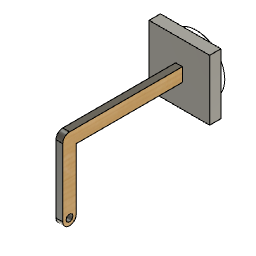
stamp1 v4 (Autodesk Fusion 360 design; units mm, degrees)
Autodesk Fusion 360 part; units mm, degrees
note: some values were not read from the file. Chosen so that the rebuilt part matches the saved one: which bodies a step acts on.
sketch "Sketch1" plane through (0, 0, 0) normal (0, 1, 0) x (1, 0, 0)
  arc A0 (0.3848, -1.12) -> (0.9072, -0.7632) centre (-0.0957, 0.1445) ccw
  arc A1 (3.1397, -0.683) -> (4.2167, 0.662) centre (1.059, 2.0869) ccw
  arc A2 (0.9072, -0.7632) -> (2.7383, -0.9246) centre (1.9676, 0.8001) ccw
  arc A3 (3.0458, -0.7511) -> (3.0474, -0.7499) centre (2.7604, -0.3405) ccw
  arc A4 (-1.811, -5.1195) -> (0.4336, -3.2886) centre (-2.5419, -1.932) ccw
  arc A5 (3.5281, -4.1281) -> (3.0649, -1.2688) centre (0.4022, -3.1674) ccw
  arc A6 (1.1624, -0.2268) -> (1.1146, 0.4041) centre (-0.173, -0.0107) ccw
  arc A7 (1.1146, 0.4041) -> (2.1699, 1.9092) centre (0.2909, 2.1041) ccw
  arc A8 (5.3391, 0.9914) -> (2.6312, 2.0198) centre (2.9441, -1.2354) ccw
  arc A9 (0.7776, 0.8933) -> (0.2074, 1.1673) centre (-0.0773, -0.1552) ccw
  arc A10 (0.2074, 1.1673) -> (-0.5684, 2.8338) centre (-1.6767, 1.304) ccw
  arc A11 (-0.9784, 3.0605) -> (-2.6817, 3.3207) centre (-2.3368, -0.1263) ccw
  arc A12 (1.811, 5.1195) -> (-0.4336, 3.2886) centre (2.5419, 1.932) ccw
  arc A13 (-0.3848, 1.12) -> (-0.9072, 0.7632) centre (0.0957, -0.1445) ccw
  arc A14 (-0.9072, 0.7632) -> (-2.7383, 0.9246) centre (-1.9676, -0.8001) ccw
  arc A15 (-3.1397, 0.683) -> (-4.2167, -0.662) centre (-1.059, -2.0869) ccw
  arc A16 (-3.5281, 4.1281) -> (-3.0649, 1.2688) centre (-0.4022, 3.1674) ccw
  arc A17 (-1.1624, 0.2268) -> (-1.1146, -0.4041) centre (0.173, 0.0107) ccw
  arc A18 (-1.1146, -0.4041) -> (-2.1699, -1.9092) centre (-0.2909, -2.1041) ccw
  arc A19 (-2.1613, -2.3776) -> (-1.535, -3.9828) centre (1.2778, -1.9605) ccw
  arc A20 (-5.3391, -0.9914) -> (-2.6312, -2.0198) centre (-2.9441, 1.2354) ccw
  arc A21 (-0.7776, -0.8933) -> (-0.2074, -1.1673) centre (0.0773, 0.1552) ccw
  arc A22 (-0.2074, -1.1673) -> (0.5684, -2.8338) centre (1.6767, -1.304) ccw
  arc A23 (0.9784, -3.0605) -> (2.6817, -3.3207) centre (2.3368, 0.1263) ccw
  arc A24 (0.5684, -2.8338) -> (0.3848, -1.12) centre (-2.2605, -2.2702) ccw
  arc A25 (-2.1699, -1.9092) -> (-0.7776, -0.8933) centre (-3.0963, 0.8225) ccw
  arc A26 (-2.7383, 0.9246) -> (-1.1624, 0.2268) centre (-0.8358, 3.0927) ccw
  arc A27 (-0.5684, 2.8338) -> (-0.3848, 1.12) centre (2.2605, 2.2702) ccw
  arc A28 (2.1699, 1.9092) -> (0.7776, 0.8933) centre (3.0963, -0.8225) ccw
  arc A29 (2.7383, -0.9246) -> (1.1624, -0.2268) centre (0.8358, -3.0927) ccw
  line L0 (6.7, -6.7) -> (-6.7, -6.7)
  line L1 (-6.7, -6.7) -> (-6.7, 6.7)
  line L2 (-6.7, 6.7) -> (6.7, 6.7)
  line L3 (6.7, 6.7) -> (6.7, -6.7)
  arc A30 (-0.6739, -1.5178) -> (0.4336, -3.2886) centre (1.5858, -1.3364) ccw
  arc A31 (0.818, -3.4693) -> (2.6817, -3.3207) centre (1.5858, -1.3364) ccw
  arc A32 (-1.811, -5.1195) -> (0.818, -3.4693) centre (-1.8093, -2.2029) ccw
  arc A33 (0.9784, -3.0605) -> (0.9775, -1.3425) centre (-1.8093, -2.2029) ccw
  arc A34 (0.9775, -1.3425) -> (3.0649, -1.2688) centre (1.9502, 0.7051) ccw
  arc A35 (3.4135, -1.0262) -> (4.2167, 0.662) centre (1.9502, 0.7051) ccw
  arc A36 (3.1397, -0.683) -> (1.6513, 0.1753) centre (1.0032, -2.6683) ccw
  arc A37 (3.5281, -4.1281) -> (3.4135, -1.0262) centre (1.0032, -2.6683) ccw
  arc A38 (1.6513, 0.1753) -> (2.6312, 2.0198) centre (0.3645, 2.0415) ccw
  arc A39 (2.5955, 2.4431) -> (1.535, 3.9828) centre (0.3645, 2.0415) ccw
  arc A40 (2.1613, 2.3776) -> (0.6739, 1.5178) centre (2.8124, -0.4654) ccw
  arc A41 (5.3391, 0.9914) -> (2.5955, 2.4431) centre (2.8124, -0.4654) ccw
  arc A42 (0.6739, 1.5178) -> (-0.4336, 3.2886) centre (-1.5858, 1.3364) ccw
  arc A43 (-0.818, 3.4693) -> (-2.6817, 3.3207) centre (-1.5858, 1.3364) ccw
  arc A44 (-0.9784, 3.0605) -> (-0.9775, 1.3425) centre (1.8093, 2.2029) ccw
  arc A45 (1.811, 5.1195) -> (-0.818, 3.4693) centre (1.8093, 2.2029) ccw
  arc A46 (-0.9775, 1.3425) -> (-3.0649, 1.2688) centre (-1.9502, -0.7051) ccw
  arc A47 (-3.4135, 1.0262) -> (-4.2167, -0.662) centre (-1.9502, -0.7051) ccw
  arc A48 (-3.1397, 0.683) -> (-1.6513, -0.1753) centre (-1.0032, 2.6683) ccw
  arc A49 (-3.5281, 4.1281) -> (-3.4135, 1.0262) centre (-1.0032, 2.6683) ccw
  arc A50 (-1.6513, -0.1753) -> (-2.6312, -2.0198) centre (-0.3645, -2.0415) ccw
  arc A51 (-2.5955, -2.4431) -> (-1.535, -3.9828) centre (-0.3645, -2.0415) ccw
  arc A52 (-2.1613, -2.3776) -> (-0.6739, -1.5178) centre (-2.8124, 0.4654) ccw
  arc A53 (-5.3391, -0.9914) -> (-2.5955, -2.4431) centre (-2.8124, 0.4654) ccw
  arc A54 (2.1613, 2.3776) -> (1.535, 3.9828) centre (-1.2778, 1.9605) ccw
  circle A55 centre (3.016, -4.229) radius 0.5219
  circle A56 centre (5.1704, 0.4975) radius 0.5219
  circle A57 centre (2.1544, 4.7264) radius 0.5219
  circle A58 centre (-3.016, 4.229) radius 0.5219
  circle A59 centre (-5.1704, -0.4975) radius 0.5219
  circle A60 centre (-2.1544, -4.7264) radius 0.5219
  circle A61 centre (0, 0) radius 5.9
  circle A62 centre (0, 0) radius 6.28
  dimension "d1" = 0.5
  dimension "d9" = 13.4
  dimension "d10" = 13.4
  dimension "d15" = 6.7
  dimension "d23" = 360
  dimension "d25" = 11.8
  dimension "d26" = 12.56
  dimension "d27" = 6.7
  constraint tangent A1 A3
  constraint tangent A2 A3
  constraint horizontal L0
  constraint perpendicular L0 L1
  constraint parallel L0 L2
  constraint parallel L1 L3
  constraint concentric A30 A31
  constraint concentric A32 A33
  constraint coincident A5.start A55
  constraint coincident A61.centre A62.centre
  constraint concentric A61 A62
  measures "d1" radius of A3
  measures "d9" distance of L1.end L2.end
  measures "d10" distance of L0.end L1.end
  measures "d15" distance of L1 A61.centre
  measures "d25" diameter of A61
  measures "d26" diameter of A62
  measures "d27" distance of L0 A61.centre
extrude "Extrude1" add sketch "Sketch1" along normal blind 1.25 contours A0 A1 A2 A3 A4 A5 A6 A7 A8 A9 A10 A11 A12 A13 A14 A15 A16 A17 A18 A19 A20 A21 A22 A23 A24 A25 A26 A27 A28 A29 A30 A31 A32 A33 A34 A35 A36 A37 A38 A39 A40 A41 A42 A43 A44 A45 A46 A47 A48 A49 A50 A51 A52 A53 A54 | A3 A29 A36 | A55 | A60 | A59 | A58 | A57 | A56 | A62 makes body 1 at (-2.3208, 0, 2.1022) makes body 1 at (3.5373, 0.8333, 4.2548) makes body 1 at (-1.6331, 0.4167, 4.7009) makes body 1 at (-4.9899, 0.4167, 0.0078) makes body 1 at (-3.5163, 0.8333, -4.3777) makes body 1 at (2.6757, 0.8333, -4.7007) makes body 1 at (5.6898, 0.4167, -0.4459) makes body 2 at (6.2722, 0.8333, 0.313)
extrude "Extrude2" add sketch "Sketch1" against normal blind 2.5 contours A0 A2 A3 A6 A7 A9 A10 A13 A14 A17 A18 A21 A22 A24 A25 A26 A27 A28 A29 | A0 A1 A2 A3 A4 A5 A6 A7 A8 A9 A10 A11 A12 A13 A14 A15 A16 A17 A18 A19 A20 A21 A22 A23 A24 A25 A26 A27 A28 A29 A30 A31 A32 A33 A34 A35 A36 A37 A38 A39 A40 A41 A42 A43 A44 A45 A46 A47 A48 A49 A50 A51 A52 A53 A54 | A3 A29 A36 | A3 A29 | A3 A36 | A55 | A60 | A59 | A58 | A57 | A56 | L0 L1 L2 L3 | A61 | A62 bodies 2 1
scale "Scale1" factor 2 about (-6.7, -2.5, 6.7) bodies 2
scale "Scale2" factor 2 about (5.9304, 2.5, -8.94) bodies 2
sketch "Sketch2" plane through (0, 2.5, 0) normal (0, 1, 0) x (-1, 0, 0)
  arc A0 (-18.4229, -0.7616) -> (-12.1191, -3.5529) centre (-10.8129, 7.911) ccw
  arc A1 (-12.1191, -3.5529) -> (-11.928, -6.0762) centre (-6.7775, -4.4173) ccw
  arc A2 (-11.928, -6.0762) -> (-16.1492, -12.0967) centre (-8.6334, -12.8762) ccw
  arc A3 (-16.1492, -12.0967) -> (-10.5798, -8.033) centre (-19.8548, -1.1699) ccw
  arc A4 (-10.5798, -8.033) -> (-8.2991, -9.1292) centre (-7.1605, -3.8393) ccw
  arc A5 (-8.2991, -9.1292) -> (-5.1958, -15.795) centre (-0.7628, -9.676) ccw
  arc A6 (-5.1958, -15.795) -> (-5.9304, -8.94) centre (-16.5115, -13.5408) ccw
  arc A7 (-5.9304, -8.94) -> (-3.8407, -7.5129) centre (-7.8526, -3.8819) ccw
  arc A8 (-3.8407, -7.5129) -> (3.4837, -8.1583) centre (0.401, -1.2597) ccw
  arc A9 (3.4837, -8.1583) -> (-2.8202, -5.367) centre (-4.1263, -16.8309) ccw
  arc A10 (-2.8202, -5.367) -> (-3.0112, -2.8437) centre (-8.1617, -4.5026) ccw
  arc A11 (-3.0112, -2.8437) -> (1.2099, 3.1767) centre (-6.3058, 3.9563) ccw
  arc A12 (1.2099, 3.1767) -> (-4.3594, -0.8869) centre (4.9156, -7.7501) ccw
  arc A13 (-4.3594, -0.8869) -> (-6.6401, 0.2092) centre (-7.7787, -5.0806) ccw
  arc A14 (-6.6401, 0.2092) -> (-9.7434, 6.8751) centre (-14.1764, 0.756) ccw
  arc A15 (-9.7434, 6.8751) -> (-9.0088, 0.0201) centre (1.5723, 4.6208) ccw
  arc A16 (-9.0088, 0.0201) -> (-11.0985, -1.407) centre (-7.0866, -5.038) ccw
  arc A17 (-11.0985, -1.407) -> (-18.4229, -0.7616) centre (-15.3402, -7.6602) ccw
sketch "Sketch3" plane through (0, -7.5, 0) normal (0, -1, 0) x (1, 0, 0)
  line L0 (-19.3304, -31.26) -> (34.2696, -31.26)
  line L1 (34.2696, -31.26) -> (34.2696, 22.34)
  line L2 (34.2696, 22.34) -> (-19.3304, 22.34)
  line L3 (-19.3304, 22.34) -> (-19.3304, -31.26)
  line L4 (10.4696, 10.54) -> (4.4696, 10.54)
  line L5 (4.4696, 10.54) -> (4.4696, -19.46)
  line L6 (4.4696, -19.46) -> (10.4696, -19.46)
  line L7 (10.4696, -19.46) -> (10.4696, 10.54)
  point P0 (7.4696, -4.46)
  dimension "d28" = 6
  dimension "d29" = 30
  constraint horizontal L4
  constraint perpendicular L4 L5
  constraint parallel L4 L6
  constraint parallel L5 L7
  measures "d28" distance of L5.end L6.end
  measures "d29" distance of L4.end L5.end
ref_plane "WorkPlane1" through (7.1696, -2.5, -4.46) normal (-1, 0, 0) x (0, 0, -1)
sketch "Sketch4" plane through (7.1696, -2.5, -4.46) normal (-1, 0, 0) x (0, 0, -1)
  line L0 (-26.8, -5) -> (26.8, -5)
  line L1 (26.8, -5) -> (26.8, 5)
  line L2 (26.8, 5) -> (-26.8, 5)
  line L3 (-26.8, 5) -> (-26.8, -5)
  line L4 (0, 5) -> (-6, 5)
  line L5 (-6, 5) -> (-6, 105)
  line L6 (6, 99) -> (6, 5)
  arc A0 (0, 111) -> (-6, 105) centre (0, 105) ccw
  line L7 (0, 111) -> (60, 111)
  line L8 (60, 99) -> (6, 99)
  circle A1 centre (60, 105) radius 3
  arc A2 (60, 99) -> (60, 111) centre (60, 105) ccw
  dimension "d31" = 6
  dimension "d32" = 100
  dimension "d37" = 60
  dimension "d38" = 12
  dimension "d39" = 12
  dimension "d40" = 6
  constraint midpoint L2 L4.start
  constraint coincident L2 L4.end
  constraint perpendicular L4 L5
  constraint coincident L2 L6.end
  constraint perpendicular L2 L6
  constraint tangent L5 A0
  constraint horizontal L7
  constraint perpendicular L6 L8
  constraint concentric A1 A2
  measures "d31" distance of L4.start L4.end
  measures "d32" distance of L4.end L5.end
  measures "d37" distance of A0.start L7.end
  measures "d38" distance of L7.end L8.start
  measures "d39" diameter of A2
  measures "d40" diameter of A1
extrude "Extrude3" add sketch "Sketch4" along normal mid plane 6 separate body contours L2 L4 L5 L6 A0 L7 L8 A2 makes body 3
